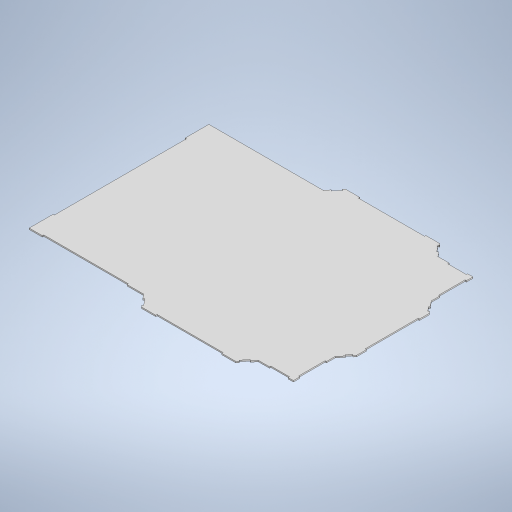
# Autodesk Inventor part: Base Plate
Saved by Autodesk Inventor 2023 (Build 270158000, 158)
## iProperties
Created: 2023-02-07
Part Number: Base Plate
Material: Generic
Document SubType Name: Modeling
Designer: cheng
Density: 1 g/cm^3
Appearance: Default
Author: cheng
Autodesk Inventor part; units mm, degrees
ref_plane "YZ Plane" through (0, 0, 0) normal (1, 0, 0) x (0, 1, 0)
ref_plane "XZ Plane" through (0, 0, 0) normal (0, 1, 0) x (-1, 0, 0)
ref_plane "XY Plane" through (0, 0, 0) normal (0, 0, 1) x (1, 0, 0)
sketch "Sketch1" plane through (0, 0, 0) normal (0, 1, 0) x (-1, 0, 0)
  line L0 (500, -340) -> (-500, -340)
  line L1 (-500, -340) -> (-500, 340)
  line L2 (-500, 340) -> (500, 340)
  line L3 (500, 340) -> (500, -340)
  line L4 (500, -340) -> (-500, 340) construction
  line L5 (-500, -340) -> (500, 340) construction
  line L6 (500, 0) -> (-500, 0) construction
  circle A0 centre (-150, 0) radius 335
  circle A1 centre (-150, 0) radius 385
  line L7 (236.875, -386.2433) -> (-536.875, -386.2433)
  line L8 (-536.875, -386.2433) -> (-536.875, 386.2433)
  line L9 (-536.875, 386.2433) -> (236.875, 386.2433)
  line L10 (236.875, 386.2433) -> (236.875, -386.2433)
  line L11 (236.875, -386.2433) -> (-536.875, 386.2433) construction
  line L12 (-536.875, -386.2433) -> (236.875, 386.2433) construction
  line L13 (236.875, -137.894) -> (28.4852, -386.2433)
  line L14 (-328.4852, -386.2433) -> (-536.875, -137.894)
  line L15 (236.875, 137.894) -> (28.4852, 386.2433)
  line L16 (-328.4852, 386.2433) -> (-536.875, 137.894)
  line L17 (500, -250) -> (495, -250)
  line L18 (495, -250) -> (495, 250)
  line L19 (495, 250) -> (500, 250)
  line L20 (500, 250) -> (500, -250)
  line L21 (500, -250) -> (495, 250) construction
  line L22 (495, -250) -> (500, 250) construction
  line L23 (130, 335) -> (450, 335)
  line L24 (450, 335) -> (450, 340)
  line L25 (450, 340) -> (130, 340)
  line L26 (130, 340) -> (130, 335)
  line L27 (130, 335) -> (450, 340) construction
  line L28 (450, 335) -> (130, 340) construction
  line L29 (-275, 381.2433) -> (-25, 381.2433)
  line L30 (-25, 381.2433) -> (-25, 386.2433)
  line L31 (-25, 386.2433) -> (-275, 386.2433)
  line L32 (-275, 386.2433) -> (-275, 381.2433)
  line L33 (-275, 381.2433) -> (-25, 386.2433) construction
  line L34 (-25, 381.2433) -> (-275, 386.2433) construction
  line L35 (-480, 335) -> (-410, 335)
  line L36 (-410, 335) -> (-410, 340)
  line L37 (-410, 340) -> (-480, 340)
  line L38 (-480, 340) -> (-480, 335)
  line L39 (-480, 335) -> (-410, 340) construction
  line L40 (-410, 335) -> (-480, 340) construction
  line L41 (-495, 215) -> (-500, 215)
  line L42 (-500, 215) -> (-500, 315)
  line L43 (-500, 315) -> (-495, 315)
  line L44 (-495, 315) -> (-495, 215)
  line L45 (-495, 215) -> (-500, 315) construction
  line L46 (-500, 215) -> (-495, 315) construction
  line L47 (30.3492, 376.2433) -> (34.1794, 379.4572)
  line L48 (34.1794, 379.4572) -> (53.463, 356.4759)
  line L49 (53.463, 356.4759) -> (49.6328, 353.262)
  line L50 (49.6328, 353.262) -> (30.3492, 376.2433)
  line L51 (-150, -386.2433) -> (-150, 383.7433) construction
  line L52 (-330.3492, 376.2433) -> (-334.1794, 379.4572)
  line L53 (-334.1794, 379.4572) -> (-353.463, 356.4759)
  line L54 (-353.463, 356.4759) -> (-349.6328, 353.262)
  line L55 (-349.6328, 353.262) -> (-330.3492, 376.2433)
  line L56 (-531.875, -100) -> (-536.875, -100)
  line L57 (-536.875, -100) -> (-536.875, 100)
  line L58 (-536.875, 100) -> (-531.875, 100)
  line L59 (-531.875, 100) -> (-531.875, -100)
  line L60 (-531.875, -100) -> (-536.875, 100) construction
  line L61 (-536.875, -100) -> (-531.875, 100) construction
  line L62 (-275, -381.2433) -> (-25, -381.2433)
  line L63 (-25, -381.2433) -> (-25, -386.2433)
  line L64 (-25, -386.2433) -> (-275, -386.2433)
  line L65 (-275, -386.2433) -> (-275, -381.2433)
  line L66 (30.3492, -376.2433) -> (34.1794, -379.4572)
  line L67 (34.1794, -379.4572) -> (53.463, -356.4759)
  line L68 (53.463, -356.4759) -> (49.6328, -353.262)
  line L69 (49.6328, -353.262) -> (30.3492, -376.2433)
  line L70 (-353.463, -356.4759) -> (-349.6328, -353.262)
  line L71 (-334.1794, -379.4572) -> (-353.463, -356.4759)
  line L72 (-349.6328, -353.262) -> (-330.3492, -376.2433)
  line L73 (-330.3492, -376.2433) -> (-334.1794, -379.4572)
  line L74 (-530.7052, -145.2469) -> (-526.875, -142.033)
  line L75 (-526.875, -142.033) -> (-514.0192, -157.3538)
  line L76 (-514.0192, -157.3538) -> (-517.8494, -160.5678)
  line L77 (-517.8494, -160.5678) -> (-530.7052, -145.2469)
  line L78 (-480, -335) -> (-410, -335)
  line L79 (-410, -335) -> (-410, -340)
  line L80 (-410, -340) -> (-480, -340)
  line L81 (-480, -340) -> (-480, -335)
  line L82 (-495, -215) -> (-500, -215)
  line L83 (-500, -215) -> (-500, -315)
  line L84 (-500, -315) -> (-495, -315)
  line L85 (-495, -315) -> (-495, -215)
  line L86 (-530.7052, 145.2469) -> (-526.875, 142.033)
  line L87 (-526.875, 142.033) -> (-514.0192, 157.3538)
  line L88 (-514.0192, 157.3538) -> (-517.8494, 160.5678)
  line L89 (-517.8494, 160.5678) -> (-530.7052, 145.2469)
  point P0 (0, 0)
  point P1 (-367.2879, -340)
  point P2 (67.2879, -340)
  point P3 (67.2879, 340)
  point P4 (-367.2879, 340)
  point P5 (-500, 181.8399)
  point P6 (-500, -181.8399)
  point P7 (497.5, 0)
  point P8 (290, 337.5)
  point P9 (-445, 337.5)
  point P10 (-497.5, 265)
  point P11 (-497.5, 315)
  point P12 (-534.375, 0)
  point P13 (-531.875, 48.9542)
  point P14 (-500, 160.3901)
  point P15 (-500, -160.3901)
  point P16 (-531.875, -48.9542)
  point P17 (-444.9271, 247.4732)
  point P18 (-444.9271, -247.4732)
  dimension "d0" = 1000
  dimension "d1" = 680
  dimension "d2" = 670
  dimension "d3" = 50
  dimension "d4" = 650
  dimension "d6" = 40
  dimension "d7" = 40
  dimension "d8" = 40
  dimension "d9" = 40
  dimension "d12" = 5
  dimension "d13" = 5
  dimension "d14" = 320
  dimension "d15" = 50
  dimension "d16" = 5
  dimension "d17" = 250
  dimension "d18" = 5
  dimension "d19" = 70
  dimension "d20" = 20
  dimension "d21" = 5
  dimension "d22" = 25
  dimension "d23" = 100
  dimension "d24" = 5
  dimension "d25" = 30
  dimension "d26" = 10
  dimension "d27" = 5
  dimension "d28" = 200
  dimension "d29" = 500
  dimension "d30" = 5
  dimension "d31" = 20
  dimension "d32" = 10
  constraints: 178 end point, 28 symmetric about line, 20 midpoint, 19 parallel, 10 perpendicular, 9 horizontal, 8 point on line, 7 collinear, 4 tangent, 2 centre point, 2 vertical, 1 coincident, 5 other
  measures "d0" distance of L0.start L0.end
  measures "d1" distance of L0.end L1.end
  measures "d2" diameter of A0
  measures "d3" radial gap between concentric circles of A0 A1
  measures "d4" distance from line of L3 A1.centre
  measures "d6" angle of L10 L13
  measures "d7" angle to the sketch y axis of L14
  measures "d8" angle to the sketch y axis of L16
  measures "d9" angle of L15 L10
  measures "d12" distance between parallel lines of L3 L18
  measures "d13" distance between parallel lines of L25 L23
  measures "d14" distance between parallel lines of L26 L24
  measures "d15" distance between parallel lines of L3 L24
  measures "d16" distance between parallel lines of L31 L29
  measures "d17" distance between parallel lines of L32 L30
  measures "d18" distance between parallel lines of L37 L35
  measures "d19" distance between parallel lines of L38 L36
  measures "d20" distance between parallel lines of L1 L38
  measures "d21" distance between parallel lines of L42 L44
  measures "d22" distance between parallel lines of L2 L43
  measures "d23" distance from line of point (-497.5, 315) L41
  measures "d24" distance between parallel lines of L15 L50
  measures "d25" distance between parallel lines of L47 L49
  measures "d26" distance from line of L9 L47.start
  measures "d27" distance of L57.end L58.end
  measures "d28" distance between parallel lines of L56 L58
  measures "d29" distance between parallel lines of L19 L17
  measures "d30" distance between parallel lines of L77 L75
  measures "d31" distance between parallel lines of L74 L76
  measures "d32" horizontal distance of L14.end L74.end
extrude "Extrusion1" add sketch "Sketch1" along normal blind 5 contours L79 L78 L81 L0 L1 L84 L85 L82 L14 | L14 A1 L0 | L0 A1 L62 L65 L7 L14 L73 L72 L70 | A1 L1 L2 L0 | L0 A1 L62 | L14 L1 A1 | A1 L13 L0 | L0 L13 L68 L69 L66 L7 L63 L62 A1 | A1 L59 L1 | L1 L14 L76 L75 L74 L8 L56 L59 A1 | L13 L10 L0 | A1 L15 L10 L13 | A1 L59 L58 L8 L16 L86 L87 L88 L1 | L1 L16 A1 | L10 L23 L24 L2 L3 L19 L18 L17 L0 | L1 L41 L44 L43 L2 L38 L35 L36 L16 | L16 L2 A1 | L15 L2 L26 L23 L10 | A1 L2 L15 | A1 L29 L2 | L2 L16 L54 L55 L52 L9 L32 L29 A1 | A1 L29 L30 L9 L15 L47 L50 L49 L2 | A0
body "Solid1"
